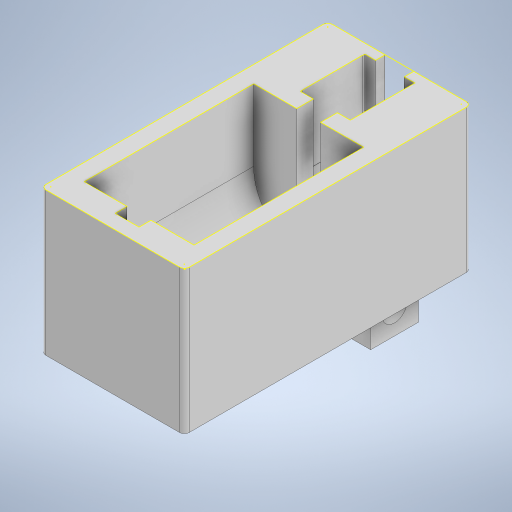
# Autodesk Inventor part: housing_V3
Saved by Autodesk Inventor 2023 (Build 270158000, 158)
## iProperties
Created: 2023-03-23
Part Number: housing_V3
Material: Generic
Document SubType Name: Modeling
Designer: caleb
Density: 1 g/cm^3
Appearance: Default
Author: caleb
## iProperties of the stored document housing_V2_3DPrint.ipt
Created: 2023-03-24
Part Number: housing_V2_3DPrint
Material: Generic
Document SubType Name: Modeling
Designer: caleb
Density: 1 g/cm^3
Appearance: Default
Author: caleb
Autodesk Inventor part; units mm, degrees
sketch "Sketch1" plane through (0, 0, 0) normal (0, 1, 0) x (-1, 0, 0)
  line L0 (-0.0661, 0.1517) -> (59.9339, 0.1517)
  line L1 (59.9339, 0.1517) -> (59.9339, -119.8483)
  line L2 (59.9339, -119.8483) -> (-0.0661, -119.8483)
  line L3 (-0.0661, -119.8483) -> (-0.0661, 0.1517)
  line L4 (29.9339, -119.8483) -> (29.9339, 0.1517)
  circle A0 centre (29.9339, -54.8547) radius 22.5
  line L5 (19.5008, -89.8484) -> (19.5008, -114.8484)
  line L6 (19.5008, -114.8484) -> (40.5008, -114.8484)
  line L7 (40.5008, -114.8484) -> (40.5008, -89.8484)
  line L8 (40.5008, -89.8484) -> (19.5008, -89.8484)
  line L9 (19.5008, -89.8484) -> (40.5008, -114.8484) construction
  line L10 (19.5008, -114.8484) -> (40.5008, -89.8484) construction
  line L11 (19.5008, -89.8484) -> (44.5008, -89.8484) construction
  line L12 (24.9546, -79.8533) -> (24.9546, -89.8533)
  line L13 (24.9546, -89.8533) -> (34.9546, -89.8533)
  line L14 (34.9546, -89.8533) -> (34.9546, -79.8533)
  line L15 (34.9546, -79.8533) -> (24.9546, -79.8533)
  line L16 (24.9546, -79.8533) -> (34.9546, -89.8533) construction
  line L17 (24.9546, -89.8533) -> (34.9546, -79.8533) construction
  line L18 (24.9546, -79.8533) -> (34.9546, -79.8533) construction
  line L19 (7.4339, -10.8533) -> (7.4339, -79.8533)
  line L20 (7.4339, -79.8533) -> (52.4339, -79.8533)
  line L21 (52.4339, -79.8533) -> (52.4339, -10.8533)
  line L22 (52.4339, -10.8533) -> (7.4339, -10.8533)
  line L23 (7.4339, -10.8533) -> (52.4339, -79.8533) construction
  line L24 (7.4339, -79.8533) -> (52.4339, -10.8533) construction
  line L25 (7.4339, -10.8533) -> (76.4339, -10.8533) construction
  line L26 (34.9339, -5.8533) -> (24.9339, -5.8533)
  line L27 (24.9339, -5.8533) -> (24.9339, -15.8533)
  line L28 (24.9339, -15.8533) -> (34.9339, -15.8533)
  line L29 (34.9339, -15.8533) -> (34.9339, -5.8533)
  line L30 (34.9339, -5.8533) -> (24.9339, -15.8533) construction
  line L31 (24.9339, -5.8533) -> (34.9339, -15.8533) construction
  point P0 (0, 0)
  point P1 (29.9339, -114.8483)
  point P2 (30.4342, -89.8533)
  point P3 (29.9546, -89.8533)
  point P4 (29.9339, -79.8533)
  point P5 (30.0136, -77.3546)
  point P6 (29.9339, -25)
  point P7 (30.0008, -102.3484)
  point P8 (29.9339, -10.8533)
  point P9 (29.9546, -84.8533)
  point P10 (29.9339, -10.8533)
  point P11 (29.9339, -45.3533)
  point P12 (34.9546, -79.8533)
  point P13 (24.9546, -79.8533)
  point P14 (24.9546, -89.8484)
  point P15 (34.9546, -89.8484)
  point P16 (34.9339, -10.8533)
  point P17 (24.9339, -10.8533)
  dimension "d0" = 60
  dimension "d1" = 120
  dimension "d2" = 45
  dimension "d3" = 5
  dimension "d4" = 25
  dimension "d6" = 12.5
  dimension "d7" = 10
  dimension "d8" = 2.5
  dimension "d9" = 22.5
  dimension "d10" = -69
  dimension "d11" = 25
  dimension "d12" = 90
  dimension "d13" = 21
  dimension "d14" = 5
  dimension "d15" = 10
  dimension "d16" = 90
  dimension "d17" = 10
  dimension "d18" = -69
  dimension "d19" = 90
  dimension "d20" = -34.5
  dimension "d21" = 45
  dimension "d42" = 10
  dimension "d43" = 10
  constraints: 64 end point, 13 parallel, 11 midpoint, 8 perpendicular, 6 point on line, 4 horizontal, 2 coincident, 1 centre point
  measures "d0" distance of L2.start L2.end
  measures "d1" distance of L1.start L2.start
  measures "d2" diameter of A0
  measures "d3" distance from line of L2 point (29.934, -114.848)
  measures "d4" distance of point (30.434, -89.853) point (29.934, -114.848)
  measures "d6" distance of point (29.934, -114.848) point (30.001, -102.348)
  measures "d7" distance of point (29.934, -79.853) point (29.955, -89.853)
  measures "d8" distance of point (30.014, -77.355) point (29.934, -79.853)
  measures "d9" distance of point (29.934, -54.855) point (30.014, -77.355)
  measures "d10" distance of point (29.934, -10.853) point (29.934, -79.853)
  measures "d11" distance of L8.end L5.end
  measures "d12" angle of L5 L11
  measures "d13" distance of L7.start L5.end
  measures "d14" distance of point (29.955, -84.853) point (29.955, -89.853)
  measures "d15" distance of L15.end L12.end
  measures "d16" angle of L12 L18
  measures "d17" distance of L14.start L12.end
  measures "d18" distance of L19.start L20.start
  measures "d19" angle of L19 L25
  measures "d20" distance of point (29.934, -79.853) point (29.934, -45.353)
  measures "d21" distance between parallel lines of L19 L21
  measures "d42" distance of L26.start L26.end
  measures "d43" distance of L27.end L26.end
extrude "Extrusion1" add sketch "Sketch1" against normal blind 60
sketch "Sketch2" plane through (0.0661, 0, -119.8483) normal (0, 0, -1) x (-1, 0, 0)
  line L0 (0, 0) -> (60, 0) projected
  line L1 (0, 0) -> (0, -60) projected
  line L2 (60, -60) -> (0, -60) projected
  line L3 (60, 0) -> (60, -60) projected
  point P0 (0.0661, 0)
  point P1 (30, -30)
ref_plane "Work Plane1" through (-19.5008, 0, -114.8484) normal (0, 0, -1) x (-1, 0, 0)
ref_plane "Work Plane2" through (-19.5008, 0, -89.8484) normal (0, 0, -1) x (-1, 0, 0)
ref_plane "Work Plane3" through (-24.9546, 0, -79.8533) normal (0, 0, -1) x (-1, 0, 0)
ref_plane "Work Plane5" through (-7.4339, 0, -5.8533) normal (0, 0, -1) x (-1, 0, 0)
ref_plane "Work Plane4" through (-7.4339, 0, -10.8533) normal (0, 0, -1) x (-1, 0, 0)
sketch "Sketch3" plane through (-19.5008, 0, -114.8484) normal (0, 0, -1) x (-1, 0, 0)
  circle A0 centre (10.433, -30) radius 10.5
  point P0 (-19.5008, 0)
  dimension "d25" = 21
  constraints: 1 centre point, 1 coincident
  measures "d25" diameter of A0
ref_plane "Work Plane6" through (-29.9339, -30, -119.8483) normal (0, 1, 0) x (1, 0, 0)
extrude "Extrusion3" cut sketch "Sketch1" against normal up to surface (30 mm away) contours L22 L29 L28 L4 | L4 L28 L27 L22 | L6 L5 L8 L12 L13 L4 | L4 L13 L14 L8 L7 L6 | L28 L29 L22 L21 A0 L4 | L4 A0 L19 L22 L27 L28 | L13 L12 L8 L4 | L4 L8 L14 L13 | A0 L4 | L4 A0 | L8 L12 L15 L4 | L4 L15 L14 L8 | A0 L21 L20 L15 L4 | L4 L15 L20 L19 A0
sketch "Sketch4" plane through (-19.5008, 0, -89.8484) normal (0, 0, -1) x (-1, 0, 0)
  circle A0 centre (10.433, -30) radius 5
  point P0 (-19.5008, 0)
  point P1 (15.4537, 0)
  point P2 (15.4537, 0)
  point P3 (15.4537, 0)
  point P4 (5.4537, 0)
  point P5 (5.4537, 0)
  point P6 (5.4537, 0)
  dimension "d30" = 10
  constraints: 1 centre point, 1 coincident
  measures "d30" diameter of A0
sketch "Sketch5" plane through (-24.9546, 0, -79.8533) normal (0, 0, -1) x (-1, 0, 0)
  circle A0 centre (4.9793, -30) radius 23
  point P0 (-24.9546, 0)
  dimension "d31" = 46
  constraints: 1 centre point, 1 coincident
  measures "d31" diameter of A0
extrude "Extrusion4" cut sketch "Sketch3" against normal up to surface (25 mm away)
ref_plane "Work Plane7" through (0.0661, 0, -117.8483) normal (0, 0, -1) x (-1, 0, 0)
extrude "Extrusion5" cut sketch "Sketch4" against normal up to surface (83.9952 mm away)
extrude "Extrusion6" cut sketch "Sketch5" against normal up to surface (69 mm away)
extrude "Extrusion7" cut sketch "Sketch4" along normal up to surface (27.9998 mm away)
fillet "Fillet1" radius 2 4 edges at (-59.9339, -30, 0.1517) (0.0661, -30, 0.1517) (0.0661, -30, -119.8483) (-59.9339, -30, -119.8483)
extrude "Extrusion8" cut sketch "Sketch1" against normal through all contours L22 L29 L28 L4 | L4 L28 L27 L22
chamfer "Chamfer1" distance 2 angle 45 4 edges at (-29.9339, -60, -10.8533) (-24.9339, -60, -13.3533) (-29.9339, -60, -15.8533) (-34.9339, -60, -13.3533)
chamfer "Chamfer2" distance 2 angle 45 3 edges at (-34.9339, -52.4499, -13.3533) (-29.9339, -53, -15.8533) (-24.9339, -52.4499, -13.3533)
fillet "Fillet2" radius 1 1 edges at (-24.9339, -30, -114.8484)
fillet "Fillet3" radius 1 1 edges at (-24.9339, -30, -10.8533)
sketch "Sketch7" plane through (-1.9339, 0, -119.8483) normal (0, 0, -1) x (-1, 0, 0)
  circle A0 centre (28, -30) radius 6 projected
  line L0 (50.5, -30) -> (33.0207, -30) projected
  line L1 (34, -30) -> (34, 0)
  line L2 (33.0207, 0) -> (33.0207, -30) projected
  line L3 (23.0207, 0) -> (5.5, 0) projected
  line L4 (34, -30) -> (22, -30)
  line L5 (22, -30) -> (22, 0)
  line L6 (22, 0) -> (34, 0)
  line L7 (34, 0) -> (34, -30)
  point P0 (-1.9339, 0)
  constraints: 10 end point, 3 parallel, 2 point on line, 1 horizontal, 1 perpendicular, 2 other
extrude "Extrusion11" cut sketch "Sketch7" against normal blind 10
sketch "Sketch8" plane through (0, -60, 0) normal (0, -1, 0) x (1, 0, 0)
  line L0 (-57.9339, -119.8483) -> (-1.9339, -119.8483) projected
  line L1 (-29.9339, -119.8483) -> (-29.9339, -109.8483)
  line L2 (-29.9339, -109.8483) -> (-21.9339, -109.8483)
  line L3 (-19.5008, -114.8484) -> (-19.5008, -89.8484) projected
  line L4 (-29.9339, -109.8483) -> (-37.6839, -109.8483)
  line L5 (-21.9339, -109.8483) -> (-37.9339, -109.8483)
  line L6 (-37.9339, -109.8483) -> (-37.9339, -89.8483)
  line L7 (-37.9339, -89.8483) -> (-21.9339, -89.8483)
  line L8 (-21.9339, -89.8483) -> (-21.9339, -109.8483)
  line L9 (-37.9339, -89.8483) -> (-47.9339, -89.8483)
  line L10 (-47.9339, -89.8483) -> (-47.9339, -109.8483)
  line L11 (-47.9339, -109.8483) -> (-37.9339, -109.8483)
  line L12 (-37.9339, -109.8483) -> (-37.9339, -89.8483)
  line L13 (-21.9339, -109.8483) -> (-11.9339, -109.8483)
  line L14 (-11.9339, -109.8483) -> (-11.9339, -89.8483)
  line L15 (-11.9339, -89.8483) -> (-21.9339, -89.8483)
  line L16 (-21.9339, -89.8483) -> (-21.9339, -109.8483)
  line L17 (-24.9339, -89.8484) -> (-34.9339, -89.8484) projected
  point P0 (0, 0)
  point P1 (-24.9546, -89.8484)
  dimension "d72" = 8
  dimension "d74" = 20
  dimension "d75" = 10
  dimension "d76" = 10
  dimension "d87" = 16
  constraints: 30 end point, 6 parallel, 4 horizontal, 4 perpendicular, 1 midpoint, 1 vertical
  measures "d72" distance of L1.end L2.end
  measures "d74" distance of L5.end L6.end
  measures "d75" distance of L11.end L10.end
  measures "d76" distance of L15.end L14.end
  measures "d87" distance of L2.end L5.end
extrude "Extrusion12" add sketch "Sketch8" along normal blind 20 contours L8 L15 L3 L13 | L3 L15 L14 L13 | L11 L10 L9 L6
sketch "Sketch9" plane through (-11.9339, -60, -89.8483) normal (1, 0, 0) x (0, 0, -1)
  line L0 (0, 0) -> (0, -20) projected
  line L1 (0, -20) -> (20, -20) projected
  line L2 (10, -20) -> (10, -10)
  circle A0 centre (10, -10) radius 3.25
  point P0 (-89.8483, 60)
  dimension "d81" = 6.5
  constraints: 2 end point, 1 centre point, 1 coincident, 1 midpoint, 1 vertical
  measures "d81" diameter of A0
extrude "Extrusion13" cut sketch "Sketch9" against normal through all
chamfer "Chamfer3" distance 2 angle 45 4 edges at (-11.9339, -70, -96.5983) (-37.9339, -70, -96.5983) (-21.9339, -70, -96.5983) (-47.9339, -70, -96.5983)
ref_plane "Work Plane8" through (-30, 0, 0) normal (1, 0, 0) x (0, 1, 0)
sketch "Sketch10" plane through (0, -60, 0) normal (0, -1, 0) x (1, 0, 0)
  line L0 (-19.4339, -89.8484) -> (-40.4339, -89.8484) projected
  line L1 (-29.9339, -89.8484) -> (-29.9339, -84.8484)
  line L2 (-29.9339, -84.8484) -> (-21.9339, -84.8484)
  line L3 (-21.9339, -109.8483) -> (-21.9339, -89.8483) projected
  line L4 (-21.9339, -84.8484) -> (-37.9339, -84.8484)
  line L5 (-37.9339, -84.8484) -> (-37.9339, -80.8484)
  line L6 (-37.9339, -80.8484) -> (-21.9339, -80.8484)
  line L7 (-21.9339, -80.8484) -> (-21.9339, -84.8484)
  point P0 (0, 0)
  point P1 (-19.5008, -89.8484)
  dimension "d89" = 5
  dimension "d90" = 4
  constraints: 12 end point, 2 parallel, 2 perpendicular, 1 horizontal, 1 midpoint, 1 vertical
  measures "d89" distance of L1.start L1.end
  measures "d90" distance of L4.end L5.end
extrude "Extrusion14" add sketch "Sketch10" along normal blind 20
sketch "Sketch11" plane through (-30, 0, 0) normal (1, 0, 0) x (0, 1, 0)
  line L0 (-80, -84.8484) -> (-80, -80.8484) projected
  line L1 (-80, -80.8484) -> (-60, -25.8989)
  line L2 (-60, -1.8483) -> (-60, -117.8483) projected
  line L3 (-80, -80.8484) -> (-21.5239, -80.8484) construction
  line L4 (-80, -80.8484) -> (-74, -80.8484)
  line L5 (-60, -80.8484) -> (-80, -80.8484) projected
  line L6 (-74, -80.8484) -> (-60, -42.3838)
  point P0 (0, 0)
  dimension "d93" = 70
  dimension "d95" = 6
  constraints: 8 end point, 3 point on line, 1 equal length, 1 horizontal
  measures "d93" angle of L3 L1
  measures "d95" distance of L0.end L4.end
extrude "Extrusion15" add sketch "Sketch11" along normal mid plane 16 contours L1 L2 L6 L4
sketch "Sketch12" plane through (-7.4339, 0, -10.8533) normal (0, 0, -1) x (-1, 0, 0)
  circle A0 centre (22.5, -30) radius 5 projected
  line L0 (27.5207, 0) -> (27.5207, -30) projected
  line L1 (27.5, -30) -> (27.5207, 0)
  line L2 (17.5207, 0) -> (17.5207, -29.5455) projected
  line L3 (27.5207, 0) -> (17.5207, 0)
  line L4 (17.5207, 0) -> (17.5, -29.9966)
  arc A1 (17.5207, -29.5455) -> (27.5, -30) centre (22.5, -30) ccw projected
  point P0 (-7.4339, 0)
  constraints: 6 end point, 2 point on circle, 1 perpendicular, 1 tangent
extrude "Extrusion16" cut sketch "Sketch12" against normal blind 5 contours A0 | A0 L2 L3 L1
sketch "Sketch13" plane through (0, 0, 0) normal (0, 1, 0) x (1, 0, 0)
  line L0 (-52.4339, 10.8533) -> (-52.4339, 79.8533) projected
  line L1 (-52.4339, 10.8533) -> (-52.9339, 10.8533)
  line L2 (-24.9339, 79.8533) -> (-7.4339, 79.8533) projected
  line L3 (-7.4339, 79.8533) -> (-6.9339, 79.8533)
  line L4 (-52.9339, 79.8533) -> (-6.9339, 79.8533)
  line L5 (-52.9339, 10.8533) -> (-6.9339, 10.8533)
  line L6 (-22, 25.8989) -> (-22, 80.8484) projected
  line L7 (-6.9339, 79.8533) -> (-7.4339, 79.8533)
  line L8 (-7.4339, 79.8533) -> (-7.4339, 10.8533) projected
  line L9 (-7.4339, 79.8533) -> (-7.4339, 10.8533)
  line L10 (-7.4339, 79.8533) -> (-7.4339, 81.8533)
  line L11 (-7.4339, 81.8533) -> (-52.4339, 81.8533)
  line L12 (-52.4339, 81.8533) -> (-52.9339, 81.8533)
  line L13 (-7.4339, 81.8533) -> (-6.9339, 81.8533)
  line L14 (-52.9339, 81.8533) -> (-52.9339, 10.8533)
  line L15 (-52.9339, 79.8533) -> (-52.9339, 10.8533) projected
  line L16 (-6.9339, 10.8533) -> (-6.9339, 81.8533)
  point P0 (0, 0)
  dimension "d100" = 0.5
  dimension "d101" = 0.5
  dimension "d104" = 2
  constraints: 24 end point, 2 parallel, 2 perpendicular, 2 point on line, 1 collinear, 1 horizontal, 1 vertical
  measures "d100" distance of L0.start L1.end
  measures "d101" distance of L2.end L3.end
  measures "d104" distance of L2.end L10.end
extrude "Extrusion17" cut sketch "Sketch13" against normal up to surface round surface about axis through (-29.9339, -30, -79.8533) along (0, 0, 1) radius 23 far side no
sketch "Sketch14" plane through (-24.9546, 0, -79.8533) normal (0, 0, 1) x (1, 0, 0)
  arc A0 (-15.4793, -30) -> (5.4537, -28.8162) centre (-4.9793, -30) ccw projected
  circle A1 centre (-4.9793, -30) radius 23
  point P0 (24.9546, 0)
  constraints: 1 centre point, 1 coincident
extrude "Extrusion19" cut sketch "Sketch14" against normal up to surface (2 mm away)
sketch "Sketch15" plane through (0, 0, 0) normal (0, 1, 0) x (1, 0, 0)
  line L0 (-19.5008, 114.8484) -> (-19.5008, 89.8484) projected
  line L1 (-19.5008, 114.8484) -> (-40.4339, 114.8484) projected
  line L2 (-40.4339, 89.8484) -> (-40.4339, 114.8484) projected
  line L3 (-40.4339, 89.8484) -> (-19.5008, 89.8484) projected
  line L4 (-19.5008, 89.8484) -> (-24.9546, 89.8484) projected
  line L5 (-19.5008, 89.8484) -> (-20.5008, 89.8484)
  line L6 (-20.5008, 89.8484) -> (-20.5008, 88.8484)
  line L7 (-20.5008, 88.8484) -> (-19.5008, 88.8484)
  line L8 (-19.5008, 88.8484) -> (-19.5008, 89.8484)
  line L9 (-40.4339, 114.8484) -> (-39.4339, 114.8484)
  line L10 (-39.4339, 114.8484) -> (-39.4339, 115.8484)
  line L11 (-39.4339, 115.8484) -> (-40.4339, 115.8484)
  line L12 (-40.4339, 115.8484) -> (-40.4339, 114.8484)
  line L13 (-40.4339, 115.8484) -> (-19.5008, 115.8484)
  line L14 (-19.5008, 115.8484) -> (-19.5008, 88.8484)
  line L15 (-19.5008, 88.8484) -> (-40.4339, 88.8484)
  line L16 (-40.4339, 88.8484) -> (-40.4339, 115.8484)
  point P0 (0, 0)
  dimension "d112" = 1
  dimension "d113" = 1
  dimension "d114" = 1
  dimension "d115" = 1
  constraints: 24 end point, 6 parallel, 3 horizontal, 3 perpendicular
  measures "d112" distance of L7.end L6.end
  measures "d113" distance of L6.end L5.end
  measures "d114" distance of L11.end L10.end
  measures "d115" distance of L10.end L9.end
extrude "Extrusion20" cut sketch "Sketch15" against normal up to surface round surface about axis through (-29.9339, -30, -114.8484) along (0, 0, 1) radius 10.5 far side no
ref_plane "Work Plane9" through (-29.9339, -30, -115.8484) normal (0, 0, 1) x (1, 0, 0)
sketch "Sketch16" plane through (-29.9339, -30, -115.8484) normal (0, 0, 1) x (1, 0, 0)
  arc A0 (-6, 8.6168) -> (-10.5, 0) centre (0, 0) ccw projected
  arc A1 (-10.5, 0) -> (10.433, 1.1838) centre (0, 0) ccw projected
  arc A2 (10.433, 1.1838) -> (6, 8.6168) centre (0, 0) ccw projected
  line L0 (6, 8.6168) -> (6, 0) projected
  arc A3 (-6, 0) -> (6, 0) centre (0, 0) ccw projected
  line L1 (-6, 0) -> (-6, 8.6168) projected
  arc A4 (10.433, 1.1838) -> (6, 8.6168) centre (0, 0) ccw projected
  circle A5 centre (0, 0) radius 10.5
  point P0 (29.9339, 30)
  constraints: 1 coincident, 3 other
extrude "Extrusion21" cut sketch "Sketch16" along normal up to surface (27 mm away)
sketch "Sketch17" plane through (0, 0, 0) normal (0, 1, 0) x (1, 0, 0)
  line L0 (-34.9546, 88.8484) -> (-40.4339, 88.8484) projected
  line L1 (-40.4339, 88.8484) -> (-40.4339, 89.8484) projected
  line L2 (-40.4339, 89.8484) -> (-40.5008, 89.8484) projected
  line L3 (-40.5008, 89.8484) -> (-40.5008, 114.8484) projected
  line L4 (-40.5008, 114.8484) -> (-40.4339, 114.8484) projected
  line L5 (-40.4339, 114.8484) -> (-40.4339, 115.8484) projected
  line L6 (-40.4339, 115.8484) -> (-35.9339, 115.8484) projected
  line L7 (-35.9339, 115.8484) -> (-35.9339, 119.8483) projected
  line L8 (-35.9339, 119.8483) -> (-57.9339, 119.8483) projected
  arc A0 (-57.9339, 119.8483) -> (-59.9339, 117.8483) centre (-57.9339, 117.8483) ccw projected
  line L9 (-59.9339, 117.8483) -> (-59.9339, 1.8483) projected
  arc A1 (-59.9339, 1.8483) -> (-57.9339, -0.1517) centre (-57.9339, 1.8483) ccw projected
  line L10 (-57.9339, -0.1517) -> (-1.9339, -0.1517) projected
  arc A2 (-1.9339, -0.1517) -> (0.0661, 1.8483) centre (-1.9339, 1.8483) ccw projected
  line L11 (0.0661, 1.8483) -> (0.0661, 117.8483) projected
  arc A3 (0.0661, 117.8483) -> (-1.9339, 119.8483) centre (-1.9339, 117.8483) ccw projected
  line L12 (-1.9339, 119.8483) -> (-23.9339, 119.8483) projected
  line L13 (-23.9339, 119.8483) -> (-23.9339, 115.8484) projected
  line L14 (-23.9339, 115.8484) -> (-19.5008, 115.8484) projected
  line L15 (-19.5008, 115.8484) -> (-19.5008, 88.8484) projected
  line L16 (-19.5008, 88.8484) -> (-24.9546, 88.8484) projected
  line L17 (-24.9546, 88.8484) -> (-24.9546, 81.8533) projected
  line L18 (-24.9546, 81.8533) -> (-6.9339, 81.8533) projected
  line L19 (-6.9339, 81.8533) -> (-6.9339, 10.8533) projected
  line L20 (-6.9339, 10.8533) -> (-24.9546, 10.8533) projected
  line L21 (-24.9546, 10.8533) -> (-24.9546, 5.8533) projected
  line L22 (-24.9546, 5.8533) -> (-34.9546, 5.8533) projected
  line L23 (-34.9546, 10.8533) -> (-34.9546, 5.8533) projected
  line L24 (-34.9546, 10.8533) -> (-52.9339, 10.8533) projected
  line L25 (-52.9339, 10.8533) -> (-52.9339, 81.8533) projected
  line L26 (-52.9339, 81.8533) -> (-34.9546, 81.8533) projected
  line L27 (-34.9546, 81.8533) -> (-34.9546, 88.8484) projected
  line L28 (-35.9339, 119.8483) -> (-23.9339, 119.8483) projected
  point P0 (0, 0)
equation "\"d4\" = d11"
equation "\"d6\" = 0.5 * d4"
equation "\"d7\" = d15"
equation "\"d9\" = 0.5 * d2"
equation "\"d14\" = 0.5 * d7"
equation "\"d18\" = d10"
equation "\"d20\" = 0.5 * d10"
equation "\"d21\" = d2"
body "Solid1"
